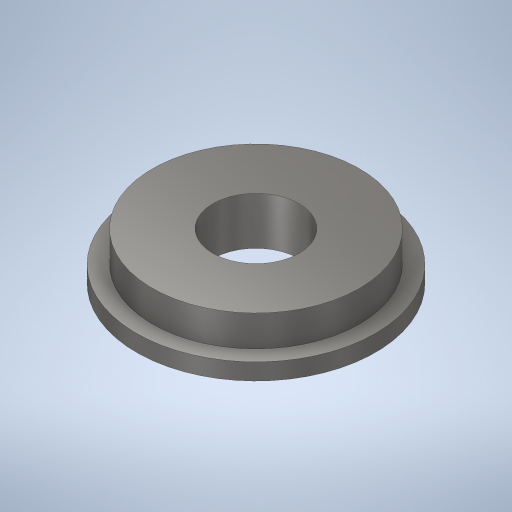
# Autodesk Inventor part: 0.1875
Saved by Autodesk Inventor 2023.3 (Build 273359000, 359)
## iProperties
Created: 2024-01-28
Part Number: 0.1875
Material: Steel
Document SubType Name: Modeling
Designer: mavericks
Density: 7.85 g/cm^3
Appearance: Semi-Polished
Author: mavericks
Autodesk Inventor part; units mm, degrees
ref_plane "YZ Plane" through (0, 0, 0) normal (1, 0, 0) x (0, 1, 0)
ref_plane "XZ Plane" through (0, 0, 0) normal (0, 1, 0) x (-1, 0, 0)
ref_plane "XY Plane" through (0, 0, 0) normal (0, 0, 1) x (1, 0, 0)
sketch "Sketch1" plane through (0, 0, 0) normal (0, 1, 0) x (-1, 0, 0)
  circle A0 centre (0, 0) radius 10.9855
  dimension "d0" = 21.971
  constraints: 1 centre point, 1 coincident
  measures "d0" diameter of A0
extrude "Extrusion1" add sketch "Sketch1" along normal blind 5.969
sketch "Sketch2" plane through (0, 5.969, 0) normal (0, 1, 0) x (1, 0, 0)
  circle A0 centre (0, 0) radius 9.525
  circle A1 centre (0, 0) radius 10.9855 projected
  circle A2 centre (0, 0) radius 10.9855 projected
  dimension "d3" = 19.05
  constraints: 1 centre point, 1 coincident
  measures "d3" diameter of A0
extrude "Extrusion2" cut sketch "Sketch2" against normal blind 4.445
sketch "Sketch3" plane through (0, 5.969, 0) normal (0, 1, 0) x (1, 0, 0)
  point P0 (0, 0)
hole "Hole1" at (0, 5.969, 0) direction (0, -1, 0) diameter 7.9375 end through all counterbore diameter 24.6126 counterbore depth 1.5875
body "Solid1"
